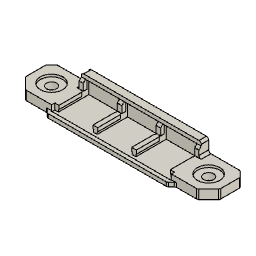
WAGO 221-413 3x3 Vertical Mount (Autodesk Fusion 360 design; units mm, degrees)
Autodesk Fusion 360 part; units mm, degrees
sketch "Sketch1" plane through (0, 0, 0) normal (0, 0, 1) x (1, 0, 0)
  line L0 (32.125, 6.1) -> (-32.125, 6.1)
  line L1 (-32.125, 6.1) -> (-32.125, -6.1)
  line L2 (-32.125, -6.1) -> (32.125, -6.1)
  line L3 (32.125, -6.1) -> (32.125, 6.1)
  line L4 (32.125, 6.1) -> (-32.125, -6.1) construction
  line L5 (-32.125, 6.1) -> (32.125, -6.1) construction
  dimension "d1" = 12.2
  dimension "d2" = 64.25
  constraint horizontal L0
  constraint perpendicular L0 L1
  constraint parallel L0 L2
  constraint parallel L1 L3
  constraint coincident L4 origin
  constraint coincident L5 origin
  measures "d1" distance of L0.start L2.end
  measures "d2" distance of L0.start L0.end
extrude "Extrude1" add sketch "Sketch1" along normal blind 22.25
sketch "Sketch2" plane through (0, 0, 22.25) normal (0, 0, 1) x (-1, 0, 0)
  line L0 (-32.125, 6.1) -> (-32.125, -6.1)
  line L1 (-32.125, -6.1) -> (32.125, -6.1)
  line L2 (32.125, -6.1) -> (32.125, 6.1)
  line L3 (32.125, 6.1) -> (-32.125, 6.1)
  line L4 (30.125, -6.1) -> (11.375, -6.1)
  line L5 (11.375, -6.1) -> (11.375, 4.1)
  line L6 (11.375, 4.1) -> (30.125, 4.1)
  line L7 (30.125, 4.1) -> (30.125, -6.1)
  line L8 (9.375, -6.1) -> (-9.375, -6.1)
  line L9 (-9.375, -6.1) -> (-9.375, 4.1)
  line L10 (-9.375, 4.1) -> (9.375, 4.1)
  line L11 (9.375, 4.1) -> (9.375, -6.1)
  line L12 (-11.375, -6.1) -> (-30.125, -6.1)
  line L13 (-30.125, -6.1) -> (-30.125, 4.1)
  line L14 (-30.125, 4.1) -> (-11.375, 4.1)
  line L15 (-11.375, 4.1) -> (-11.375, -6.1)
  dimension "d5" = 2
  dimension "d6" = 2
  dimension "d7" = 2
  dimension "d8" = 2
  dimension "d11" = 2
  constraint horizontal L4
  constraint vertical L5
  constraint horizontal L6
  constraint vertical L7
  constraint coincident L1 L4.start
  constraint horizontal L8
  constraint vertical L9
  constraint horizontal L10
  constraint vertical L11
  constraint coincident L1 L8.start
  constraint horizontal L12
  constraint vertical L13
  constraint horizontal L14
  constraint vertical L15
  constraint coincident L1 L12.start
  constraint equal L6 L10
  constraint equal L10 L14
  constraint equal L9 L15
  constraint equal L5 L11
  measures "d5" distance of L1.end L4.start
  measures "d6" distance of L0.end L12.end
  measures "d7" distance of L4.end L8.start
  measures "d8" distance of L8.end L12.start
  measures "d11" distance of L3 L13.end
extrude "Extrude2" cut sketch "Sketch2" against normal blind 20.25 contours L1 L12 L13 L14 L15 | L1 L4 L5 L6 L7 | L1 L8 L9 L10 L11
sketch "Sketch3" plane through (0, 0, 2) normal (0, 0, 1) x (-1, 0, 0)
  line L0 (-11.375, 4.1) -> (-30.125, 4.1)
  line L1 (-30.125, 4.1) -> (-30.125, -6.1)
  line L2 (-30.125, -6.1) -> (-11.375, -6.1)
  line L3 (-11.375, -6.1) -> (-11.375, 4.1)
  line L4 (9.375, 4.1) -> (-9.375, 4.1)
  line L5 (-9.375, 4.1) -> (-9.375, -6.1)
  line L6 (-9.375, -6.1) -> (9.375, -6.1)
  line L7 (9.375, -6.1) -> (9.375, 4.1)
  line L8 (30.125, 4.1) -> (11.375, 4.1)
  line L9 (11.375, 4.1) -> (11.375, -6.1)
  line L10 (11.375, -6.1) -> (30.125, -6.1)
  line L11 (30.125, -6.1) -> (30.125, 4.1)
  line L12 (30.125, -6.1) -> (-30.125, -6.1)
  line L13 (-30.125, -6.1) -> (-30.125, -4.1)
  line L14 (-30.125, -4.1) -> (30.125, -4.1)
  line L15 (30.125, -4.1) -> (30.125, -6.1)
  dimension "d12" = 2
  constraint horizontal L12
  constraint vertical L13
  constraint horizontal L14
  constraint vertical L15
  constraint coincident L1 L13.end
  constraint coincident L10.end L11.start
  measures "d12" distance of L1.end L13.end
extrude "Extrude3" add sketch "Sketch3" along normal blind 2 contours L1 L2 L3 L12 L13 L14 | L5 L6 L7 L12 L14 | L9 L10 L11 L12 L14 L15
sketch "Sketch4" plane through (0, 0, 22.25) normal (0, 0, 1) x (-1, 0, 0)
  line L0 (-11.375, 4.1) -> (-11.375, -6.1)
  line L1 (-11.375, -6.1) -> (-9.375, -6.1)
  line L2 (-9.375, -6.1) -> (-9.375, 4.1)
  line L3 (-9.375, 4.1) -> (9.375, 4.1)
  line L4 (9.375, 4.1) -> (9.375, -6.1)
  line L5 (9.375, -6.1) -> (11.375, -6.1)
  line L6 (11.375, -6.1) -> (11.375, 4.1)
  line L7 (11.375, 4.1) -> (30.125, 4.1)
  line L8 (30.125, 4.1) -> (30.125, -6.1)
  line L9 (30.125, -6.1) -> (32.125, -6.1)
  line L10 (32.125, -6.1) -> (32.125, 6.1)
  line L11 (32.125, 6.1) -> (-32.125, 6.1)
  line L12 (-32.125, 6.1) -> (-32.125, -6.1)
  line L13 (-32.125, -6.1) -> (-30.125, -6.1)
  line L14 (-30.125, -6.1) -> (-30.125, 4.1)
  line L15 (-30.125, 4.1) -> (-11.375, 4.1)
  line L16 (32.125, 4.1) -> (-32.125, 4.1)
  constraint coincident L10 L16.start
  constraint coincident L12 L16.end
  constraint perpendicular L12 L16
  constraint coincident L7.end L16
extrude "Extrude4" cut sketch "Sketch4" against normal blind 4 contours L0 L1 L2 L16 | L12 L13 L14 L16 | L4 L5 L6 L16 | L8 L9 L10 L16
sketch "Sketch5" plane through (0, 0, 18.25) normal (0, 0, 1) x (-1, 0, 0)
  line L0 (11.375, -6.1) -> (11.375, 4.1)
  line L1 (11.375, 4.1) -> (9.375, 4.1)
  line L2 (9.375, 4.1) -> (9.375, -6.1)
  line L3 (9.375, -6.1) -> (11.375, -6.1)
  line L4 (-30.125, -6.1) -> (-30.125, 4.1)
  line L5 (-30.125, 4.1) -> (-32.125, 4.1)
  line L6 (-32.125, 4.1) -> (-32.125, -6.1)
  line L7 (-32.125, -6.1) -> (-30.125, -6.1)
  line L8 (-9.375, -6.1) -> (-9.375, 4.1)
  line L9 (-9.375, 4.1) -> (-11.375, 4.1)
  line L10 (-11.375, 4.1) -> (-11.375, -6.1)
  line L11 (-11.375, -6.1) -> (-9.375, -6.1)
  line L12 (32.125, 4.1) -> (30.125, 4.1)
  line L13 (30.125, 4.1) -> (30.125, -6.1)
  line L14 (30.125, -6.1) -> (32.125, -6.1)
  line L15 (32.125, -6.1) -> (32.125, 4.1)
  line L16 (32.125, -6.1) -> (-32.125, -6.1)
  line L17 (-32.125, -6.1) -> (-32.125, 0.85)
  line L18 (-32.125, 0.85) -> (32.125, 0.85)
  line L19 (32.125, 0.85) -> (32.125, -6.1)
  dimension "d17" = 3.25
  constraint horizontal L16
  constraint vertical L17
  constraint horizontal L18
  constraint vertical L19
  constraint coincident L6 L17.end
  constraint coincident L14.end L15.start
  measures "d17" distance of L5.end L17.end
extrude "Extrude5" cut sketch "Sketch5" against normal blind 13 contours L0 L2 L3 L16 L18 | L13 L14 L15 L16 L18 L19 | L8 L10 L11 L16 L18 | L4 L6 L7 L16 L17 L18
sketch "Sketch6" plane through (0, 0, 22.25) normal (0, 0, 1) x (-1, 0, 0)
  line L0 (-32.125, 4.1) -> (32.125, 4.1)
  line L1 (32.125, 4.1) -> (32.125, 6.1)
  line L2 (32.125, 6.1) -> (-32.125, 6.1)
  line L3 (-32.125, 6.1) -> (-32.125, 4.1)
  line L4 (32.125, 6.1) -> (-32.125, 6.1)
  line L5 (-32.125, 6.1) -> (-32.125, 3.6)
  line L6 (-32.125, 3.6) -> (32.125, 3.6)
  line L7 (32.125, 3.6) -> (32.125, 6.1)
  dimension "d20" = 2.5
  constraint horizontal L4
  constraint vertical L5
  constraint horizontal L6
  constraint vertical L7
  constraint coincident L1.end L2.start
  constraint collinear L3 L5
  measures "d20" distance of L2.end L5.end
extrude "Extrude6" add sketch "Sketch6" against normal blind 2 contours L0 L5 L6 L7
sketch "Sketch7" plane through (0, 0, 18.25) normal (0, 0, 1) x (-1, 0, 0)
  line L0 (9.375, 0.85) -> (11.375, 0.85)
  line L1 (11.375, 0.85) -> (11.375, 4.1) construction
  line L2 (11.375, 4.1) -> (9.375, 4.1)
  line L3 (9.375, 4.1) -> (9.375, 0.85) construction
  line L4 (11.625, 0.85) -> (9.125, 0.85)
  line L5 (9.125, 0.85) -> (9.125, 2.85)
  line L6 (9.125, 2.85) -> (11.625, 2.85)
  line L7 (11.625, 2.85) -> (11.625, 0.85)
  line L8 (-9.125, 0.85) -> (-11.625, 0.85)
  line L9 (-11.625, 0.85) -> (-11.625, 2.85)
  line L10 (-11.625, 2.85) -> (-9.125, 2.85)
  line L11 (-9.125, 2.85) -> (-9.125, 0.85)
  line L12 (32.125, 0.85) -> (29.875, 0.85)
  line L13 (29.875, 0.85) -> (29.875, 2.85)
  line L14 (29.875, 2.85) -> (32.125, 2.85)
  line L15 (32.125, 2.85) -> (32.125, 0.85)
  line L16 (-29.875, 0.85) -> (-32.125, 0.85)
  line L17 (-32.125, 0.85) -> (-32.125, 2.85)
  line L18 (-32.125, 2.85) -> (-29.875, 2.85)
  line L19 (-29.875, 2.85) -> (-29.875, 0.85)
  line L20 (30.125, 0.85) -> (32.125, 0.85)
  line L21 (32.125, 0.85) -> (32.125, 4.1)
  line L22 (32.125, 4.1) -> (30.125, 4.1)
  line L23 (30.125, 4.1) -> (30.125, 0.85) construction
  line L24 (-11.375, 0.85) -> (-9.375, 0.85)
  line L25 (-9.375, 0.85) -> (-9.375, 4.1) construction
  line L26 (-9.375, 4.1) -> (-11.375, 4.1)
  line L27 (-11.375, 4.1) -> (-11.375, 0.85) construction
  line L28 (-32.125, 0.85) -> (-30.125, 0.85)
  line L29 (-30.125, 0.85) -> (-30.125, 4.1) construction
  line L30 (-30.125, 4.1) -> (-32.125, 4.1)
  line L31 (-32.125, 4.1) -> (-32.125, 0.85)
  dimension "d23" = 2.25
  dimension "d24" = 2.5
  dimension "d25" = 2
  constraint horizontal L4
  constraint vertical L5
  constraint horizontal L6
  constraint vertical L7
  constraint horizontal L8
  constraint vertical L9
  constraint horizontal L10
  constraint vertical L11
  constraint horizontal L12
  constraint vertical L13
  constraint horizontal L14
  constraint vertical L15
  constraint horizontal L16
  constraint vertical L17
  constraint horizontal L18
  constraint vertical L19
  constraint equal L12 L16
  constraint equal L4 L8
  constraint equal L7 L13
  constraint equal L5 L9
  constraint equal L9 L19
  constraint coincident L12.start L15.end
  constraint coincident L16.end L17.start
  constraint midpoint L0 L4
  constraint midpoint L8 L24
  measures "d23" distance of L12.start L12.end
  measures "d24" distance of L4.start L4.end
  measures "d25" distance of L12.start L14.end
extrude "Extrude7" add sketch "Sketch7" against normal blind 12.25
sketch "Sketch8" plane through (0, 0, 5.25) normal (0, 0, 1) x (-1, 0, 0)
  line L0 (11.375, -6.1) -> (11.375, 0.85) construction
  line L1 (11.375, 0.85) -> (9.375, 0.85) construction
  line L2 (9.375, 0.85) -> (9.375, -6.1) construction
  line L3 (9.375, -6.1) -> (11.375, -6.1) construction
  line L4 (30.125, 0.85) -> (30.125, -6.1) construction
  line L5 (30.125, -6.1) -> (32.125, -6.1) construction
  line L6 (32.125, -6.1) -> (32.125, 0.85) construction
  line L7 (32.125, 0.85) -> (30.125, 0.85) construction
  line L8 (-30.125, -6.1) -> (-30.125, 0.85) construction
  line L9 (-30.125, 0.85) -> (-32.125, 0.85) construction
  line L10 (-32.125, 0.85) -> (-32.125, -6.1) construction
  line L11 (-32.125, -6.1) -> (-30.125, -6.1) construction
  line L12 (-11.375, -6.1) -> (-11.375, -4.1) construction
  line L13 (-11.375, -4.1) -> (-30.125, -4.1) construction
  line L14 (-30.125, -4.1) -> (-30.125, -6.1) construction
  line L15 (-30.125, -6.1) -> (-11.375, -6.1) construction
  line L16 (32.125, -6.1) -> (-32.125, -6.1)
  line L17 (-32.125, -6.1) -> (-32.125, -4.1)
  line L18 (-32.125, -4.1) -> (32.125, -4.1)
  line L19 (32.125, -4.1) -> (32.125, -6.1)
  constraint horizontal L16
  constraint vertical L17
  constraint horizontal L18
  constraint vertical L19
  constraint coincident L10 L17.end
  constraint coincident L5.end L6.start
  constraint coincident L13.end L18
extrude "Extrude8" cut sketch "Sketch8" against normal up to surface (1.25 mm away)
sketch "Sketch9" plane through (0, 0, 5.25) normal (0, 0, 1) x (-1, 0, 0)
  line L0 (9.375, -4.1) -> (11.375, -4.1)
  line L1 (11.375, -4.1) -> (11.375, 0.85) construction
  line L2 (11.375, 0.85) -> (9.375, 0.85)
  line L3 (9.375, 0.85) -> (9.375, -4.1) construction
  line L4 (-32.125, -6.1) -> (32.125, -6.1)
  line L5 (32.125, -6.1) -> (32.125, -4.1)
  line L6 (32.125, -4.1) -> (30.125, -4.1)
  line L7 (30.125, -4.1) -> (11.375, -4.1)
  line L8 (11.375, -4.1) -> (9.375, -4.1)
  line L9 (9.375, -4.1) -> (-9.375, -4.1)
  line L10 (-9.375, -4.1) -> (-11.375, -4.1)
  line L11 (-11.375, -4.1) -> (-30.125, -4.1)
  line L12 (-30.125, -4.1) -> (-32.125, -4.1)
  line L13 (-32.125, -4.1) -> (-32.125, -6.1)
  line L14 (32.125, -4.1) -> (29.875, -4.1)
  line L15 (29.875, -4.1) -> (29.875, 0.85)
  line L16 (29.875, 0.85) -> (32.125, 0.85)
  line L17 (32.125, 0.85) -> (32.125, -4.1)
  line L18 (11.625, -4.1) -> (9.125, -4.1)
  line L19 (9.125, -4.1) -> (9.125, 0.85)
  line L20 (9.125, 0.85) -> (11.625, 0.85)
  line L21 (11.625, 0.85) -> (11.625, -4.1)
  line L22 (-9.125, -4.1) -> (-11.625, -4.1)
  line L23 (-11.625, -4.1) -> (-11.625, 0.85)
  line L24 (-11.625, 0.85) -> (-9.125, 0.85)
  line L25 (-9.125, 0.85) -> (-9.125, -4.1)
  line L26 (-32.125, -4.1) -> (-29.875, -4.1)
  line L27 (-29.875, -4.1) -> (-29.875, 0.85)
  line L28 (-29.875, 0.85) -> (-32.125, 0.85)
  line L29 (-32.125, 0.85) -> (-32.125, -4.1)
  line L30 (11.375, 2.85) -> (11.375, 4.1)
  line L31 (11.375, 4.1) -> (9.375, 4.1)
  line L32 (9.375, 4.1) -> (9.375, 2.85)
  line L33 (9.375, 2.85) -> (9.125, 2.85)
  line L34 (9.125, 2.85) -> (9.125, 0.85)
  line L35 (9.125, 0.85) -> (11.625, 0.85)
  line L36 (11.625, 0.85) -> (11.625, 2.85)
  line L37 (11.625, 2.85) -> (11.375, 2.85)
  line L38 (29.875, 0.85) -> (32.125, 0.85)
  constraint horizontal L14
  constraint vertical L15
  constraint horizontal L16
  constraint vertical L17
  constraint coincident L5.end L6.start
  constraint horizontal L18
  constraint vertical L19
  constraint horizontal L20
  constraint vertical L21
  constraint coincident L7 L18.start
  constraint horizontal L22
  constraint vertical L23
  constraint horizontal L24
  constraint vertical L25
  constraint coincident L9 L22.start
  constraint horizontal L26
  constraint vertical L27
  constraint horizontal L28
  constraint vertical L29
  constraint coincident L12.end L13.start
  constraint equal L20 L35
  constraint midpoint L0 L18
  constraint midpoint L10 L22
  constraint equal L20 L24
  constraint equal L23 L27
  constraint equal L15 L21
  constraint equal L19 L25
  constraint equal L16 L28
  constraint equal L16 L38
  constraint equal L1 L21
extrude "Extrude9" add sketch "Sketch9" against normal blind 2 contours L0 L2 L7 L8 L9 L18 L19 L20 L21 L35 | L9 L10 L11 L22 L23 L24 L25 | L6 L7 L14 L15 L16 L17 L38 | L11 L12 L26 L27 L28 L29
chamfer "Chamfer1" distance 1.25 angle 45 4 edges at (-31, 4.1, 5.25) (-10.375, 4.1, 5.25) (10.375, 4.1, 5.25) (31, 4.1, 5.25)
move_body "Move1" bodies 1 to x (1, 0, 0) y (0, 0, 1) z (0, -1, 0) at (0, 0, 0)
sketch "Sketch10" plane through (0, 0, -6.1) normal (0, 0, -1) x (1, 0, 0)
  line L0 (-32.125, 0) -> (32.125, 0)
  line L1 (32.125, 0) -> (32.125, 22.25)
  line L2 (32.125, 22.25) -> (-32.125, 22.25)
  line L3 (-32.125, 22.25) -> (-32.125, 0)
  line L4 (32.125, 0) -> (52.125, 0)
  line L5 (52.125, 0) -> (52.125, 20)
  line L6 (52.125, 20) -> (32.125, 20)
  line L7 (32.125, 20) -> (32.125, 0)
  line L8 (-32.125, 0) -> (-52.125, 0)
  line L9 (-52.125, 0) -> (-52.125, 20)
  line L10 (-52.125, 20) -> (-32.125, 20)
  line L11 (-32.125, 20) -> (-32.125, 0)
  line L12 (32.125, 20) -> (52.125, 0) construction
  line L13 (-52.125, 0) -> (-32.125, 20) construction
  circle A0 centre (42.125, 10) radius 2.7
  circle A1 centre (-42.125, 10) radius 2.7
  dimension "d34" = 20
  dimension "d35" = 5.4
  constraint horizontal L4
  constraint vertical L5
  constraint horizontal L6
  constraint vertical L7
  constraint coincident L0.end L1.start
  constraint horizontal L8
  constraint vertical L9
  constraint horizontal L10
  constraint vertical L11
  constraint coincident L0.start L3.end
  constraint equal L5 L9
  constraint equal L5 L6
  constraint equal L9 L10
  constraint midpoint L12 A0.centre
  constraint midpoint L13 A1.centre
  constraint equal A0 A1
  measures "d34" distance of L4.end L5.end
  measures "d35" diameter of A0
extrude "Extrude10" add sketch "Sketch10" against normal up to surface (5.25 mm away) contours L3 L8 L9 L10 L11 | L1 L4 L5 L6 L7
sketch "Sketch11" plane through (0, 0, -0.85) normal (0, 0, 1) x (-1, 0, 0)
  circle A0 centre (-42.125, 10) radius 2.7
  line L0 (-32.125, 5.25) -> (-30.125, 5.25)
  line L1 (-30.125, 5.25) -> (-30.125, 6)
  line L2 (-30.125, 6) -> (-29.875, 6)
  line L3 (-29.875, 6) -> (-29.875, 18.25)
  line L4 (-29.875, 18.25) -> (-32.125, 18.25)
  line L5 (-32.125, 18.25) -> (-32.125, 20)
  line L6 (-32.125, 20) -> (-52.125, 20)
  line L7 (-52.125, 20) -> (-52.125, 0)
  line L8 (-52.125, 0) -> (-32.125, 0)
  line L9 (-32.125, 0) -> (-32.125, 5.25)
  circle A1 centre (42.125, 10) radius 2.7
  line L10 (30.125, 6) -> (30.125, 5.25)
  line L11 (30.125, 5.25) -> (32.125, 5.25)
  line L12 (32.125, 5.25) -> (32.125, 0)
  line L13 (32.125, 0) -> (52.125, 0)
  line L14 (52.125, 0) -> (52.125, 20)
  line L15 (52.125, 20) -> (32.125, 20)
  line L16 (32.125, 20) -> (32.125, 18.25)
  line L17 (32.125, 18.25) -> (29.875, 18.25)
  line L18 (29.875, 18.25) -> (29.875, 6)
  line L19 (29.875, 6) -> (30.125, 6)
  circle A2 centre (42.125, 10) radius 6
  circle A3 centre (-42.125, 10) radius 6
  dimension "d38" = 12
  dimension "d39" = 12
  constraint concentric A1 A2
  constraint concentric A0 A3
  measures "d38" diameter of A2
  measures "d39" diameter of A3
extrude "Extrude11" cut sketch "Sketch11" against normal up to surface (1.25 mm away) contours A2 | A3
sketch "Sketch12" plane through (0, 0, -6.1) normal (0, 0, -1) x (1, 0, 0)
  circle A0 centre (-42.125, 10) radius 2.7
  circle A1 centre (42.125, 10) radius 2.7
  line L0 (52.125, 0) -> (52.125, 20)
  line L1 (52.125, 20) -> (32.125, 20)
  line L2 (32.125, 20) -> (32.125, 22.25)
  line L3 (32.125, 22.25) -> (-32.125, 22.25)
  line L4 (-32.125, 22.25) -> (-32.125, 20)
  line L5 (-32.125, 20) -> (-52.125, 20)
  line L6 (-52.125, 20) -> (-52.125, 0)
  line L7 (-52.125, 0) -> (52.125, 0)
  line L8 (-32.125, 22.25) -> (-34.375, 20)
  line L9 (32.125, 22.25) -> (34.375, 20)
  dimension "d44" = 45
  dimension "d45" = 45
  constraint coincident L3.end L4.start
  constraint coincident L5 L8.end
  constraint coincident L2.end L3.start
  constraint coincident L1 L9.end
  measures "d44" angle of L5 L8
  measures "d45" angle of L1 L9
extrude "Extrude12" add sketch "Sketch12" against normal up to surface (2.5 mm away) contours L1 L2 L9 | L4 L5 L8
chamfer "Chamfer3" distance 3 angle 45 2 edges at (52.125, 0, -3.475) (-52.125, 0, -3.475)
chamfer "Chamfer3" distance 6 angle 45 2 edges at (52.125, -20, -3.475) (-52.125, -20, -3.475)
fillet "Fillet2" radius 1.2 16 edges at (46.125, -20, -3.475) (52.125, -14, -3.475) (52.125, -3, -3.475) (49.125, 0, -3.475) (-46.125, -20, -3.475) (-52.125, -14, -3.475) (-52.125, -3, -3.475) (-49.125, 0, -3.475) (-32.125, -2.625, -0.85) (32.125, -2.625, -0.85) (34.375, -20, -4.85) (-32.125, -22.25, -4.85) (-34.375, -20, -4.85) (32.125, -22.25, -4.85) (32.125, -2, 6.1) (-32.125, -2, 6.1)
chamfer "Chamfer2" distance 0.4 angle 45 1 faces at (-10.5426, -13.5528, -6.1)
